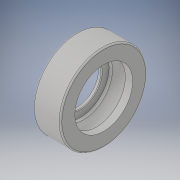
# Autodesk Inventor part: 040400DR-22-H4W(0.5)3_or
Saved by Autodesk Inventor 2024 (Build 280153000, 153)
## iProperties
Created: 2023-06-17
Part Number: 040400DR-22-H4W(0.5)3_or
Material: Generic
Catalog Web Link: www.cadenas.de
Description: DR-H or-D-Series bearings
Vendor: TOKBEARING
Document SubType Name: Modeling
Designer: psAdmin
Manufacturer: TOKBEARING
Mass: 8300 g
Surface Area: 13.8894 cm^2
Volume: 1.435 cm^3
Density: 1 g/cm^3
Appearance: PSOLRGB-175-175-175
Category: PARTsolutions
Company: TOKBEARING
PSOL_IDENT_0: {$CADENAS_DATA/23d-libs/tok_bearing/d_series_bearings/dr_h/dr_h_or.prj},191 {VTYP=3D},{NB=040400DR-2
PSOL_IDENT_1: 2-H4W(0.5)3_or},{LINA=040400DR-22-H4W(0.5)3_or},{NN=DR-H or},{DATE=16.12.2020 00:38:04},{GEOMDATE=19
PSOL_IDENT_2: .02.2013 00:00:00},{VERSION=},{LINEID=1750},{WBVAR=},{WBNUMERIC=}  {NB=040400DR-22-H4W(0.5)3_or},{LI
PSOL_IDENT_3: NA=040400DR-22-H4W(0.5)3_or},{KT=DUMMY},{IDNR=},{CODE=040400},{PN=DR-22-H4W(0.5)3},{D=22},{SD=4.0},{
PSOL_IDENT_4: W=7.0},{W1=0.5},{W1X=0.500},{W2=3},{W2X=3.000},{LOAD=196 (20)},{TYPE=12},{QTY=1.000},{GW=8.3},{BD=3.
PSOL_IDENT_5: 78},{OP=40.2862},{N=5},{R=6.415},{GP=3.64}
NB: 040400DR-22-H4W(0.5)3_or
NN: DR-H or
NT: D-Series bearings
NBSYN: $CODE.$PN._or
LINA: 040400DR-22-H4W(0.5)3_or
CATALOG: TOK, Inc
CODE: 040400
PN: DR-22-H4W(0.5)3
D: 22
SD: 4
W: 7
W1: 0.5
W2: 3
LOAD: 196 (20)
TYPE: 12
QTY: 1.000
GW: 8.3
SUPPLIER: TOKBEARING
ARTICLENO: 040400DR-22-H4W(0.5)3_or
BOMINFO: 040400DR-22-H4W(0.5)3_or
CREATOR: CADENAS GmbH
Title: 040400DR-22-H4W(0.5)3_or
Author: Cadenas PARTsolutions
Comments: D-Series bearings
Autodesk Inventor part; units mm, degrees
sketch "Sketch_2" plane through (0, 0, 0) normal (0, 0, 1) x (1, 0, 0)
  line L0 (7.15, 0) -> (0.85, 0)
  line L1 (0.5, 10.65) -> (0.5, 5.645)
  arc A0 (0.5, 5.645) -> (0.675, 5.47) centre (0.675, 5.645) ccw
  line L2 (0.675, 5.47) -> (1.325, 5.47)
  arc A1 (1.325, 5.47) -> (1.5, 5.645) centre (1.325, 5.645) ccw
  line L3 (1.5, 5.645) -> (1.5, 7.36)
  line L4 (1.5, 7.36) -> (2.3632, 7.36)
  arc A2 (5.6368, 7.36) -> (2.3632, 7.36) centre (4, 6.415) ccw
  line L5 (5.6368, 7.36) -> (7.5, 7.36)
  line L6 (7.5, 7.36) -> (7.5, 10.65)
  arc A3 (7.5, 10.65) -> (7.15, 11) centre (7.15, 10.65) ccw
  line L7 (7.15, 11) -> (0.85, 11)
  arc A4 (0.85, 11) -> (0.5, 10.65) centre (0.85, 10.65) ccw
  constraints: 16 end point, 10 point on circle, 5 centre point
revolve "Revolution1" add sketch "Sketch_2" angle 360 about axis through (7.15, 0, 0) along (1, 0, 0)
ref_plane "OR_Cage_XY" through (0, 0, 0) normal (1, 0, 0) x (0, 0, -1)
ref_plane "OR_Cage_YZ" through (0, 0, 0) normal (0, 0, -1) x (0, 1, 0)
ref_plane "OR_Cage_ZX" through (0, 0, 0) normal (0, 1, 0) x (1, 0, 0)
ref_plane "OR_IR_XY" through (0, 0, 0) normal (1, 0, 0) x (0, 0, -1)
ref_plane "OR_IR_YZ" through (0, 0, 0) normal (0, 0, -1) x (0, 1, 0)
ref_plane "OR_IR_ZX" through (0, 0, 0) normal (0, 1, 0) x (1, 0, 0)
ref_plane "OR_ball_1_XY" through (4, 6.415, 0) normal (1, 0, 0) x (0, 0, -1)
ref_plane "OR_ball_1_YZ" through (4, 6.415, 0) normal (0, 0, -1) x (0, 1, 0)
ref_plane "OR_ball_1_ZX" through (4, 6.415, 0) normal (0, 1, 0) x (1, 0, 0)
ref_plane "OR_ball_2_XY" through (4, 1.9823, 6.101) normal (1, 0, 0) x (0, 0, -1)
ref_plane "OR_ball_2_YZ" through (4, 1.9823, 6.101) normal (0, 0, -1) x (0, 1, 0)
ref_plane "OR_ball_2_ZX" through (4, 1.9823, 6.101) normal (0, 1, 0) x (1, 0, 0)
ref_plane "OR_ball_3_XY" through (4, -5.1898, 3.7706) normal (1, 0, 0) x (0, 0, -1)
ref_plane "OR_ball_3_YZ" through (4, -5.1898, 3.7706) normal (0, 0, -1) x (0, 1, 0)
ref_plane "OR_ball_3_ZX" through (4, -5.1898, 3.7706) normal (0, 1, 0) x (1, 0, 0)
ref_plane "OR_ball_4_XY" through (4, -5.1898, -3.7706) normal (1, 0, 0) x (0, 0, -1)
ref_plane "OR_ball_4_YZ" through (4, -5.1898, -3.7706) normal (0, 0, -1) x (0, 1, 0)
ref_plane "OR_ball_4_ZX" through (4, -5.1898, -3.7706) normal (0, 1, 0) x (1, 0, 0)
ref_plane "OR_ball_5_XY" through (4, 1.9823, -6.101) normal (1, 0, 0) x (0, 0, -1)
ref_plane "OR_ball_5_YZ" through (4, 1.9823, -6.101) normal (0, 0, -1) x (0, 1, 0)
ref_plane "OR_ball_5_ZX" through (4, 1.9823, -6.101) normal (0, 1, 0) x (1, 0, 0)
body "Solid1"
